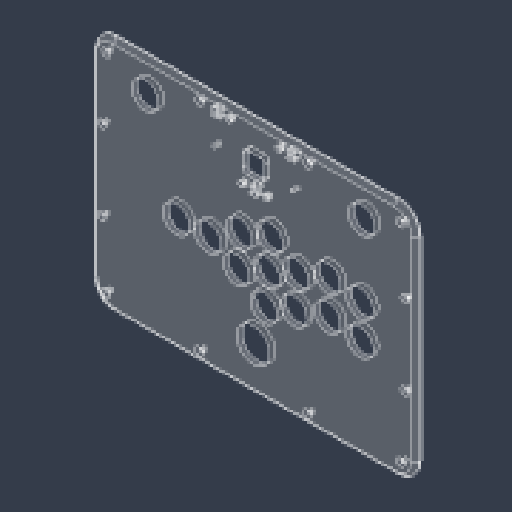
# Autodesk Inventor part: Top Plate Sanwa
Saved by Autodesk Inventor 2023.4 (Build 274418000, 418)
## iProperties
Created: 2024-02-20
Part Number: Top Plate Sanwa
Material: Polycarbonate, Clear
Document SubType Name: Modeling
Designer: JoaoSilva
Density: 1.2 g/cm^3
Appearance: Polycarbonate - Clear
Author: JoaoSilva
Autodesk Inventor part; units mm, degrees
ref_plane "YZ Plane" through (0, 0, 0) normal (1, 0, 0) x (0, 1, 0)
ref_plane "XZ Plane" through (0, 0, 0) normal (0, 1, 0) x (-1, 0, 0)
ref_plane "XY Plane" through (0, 0, 0) normal (0, 0, 1) x (1, 0, 0)
sketch "Sketch1" plane through (0, 0, 0) normal (0, 0, 1) x (1, 0, 0)
  line L0 (-150, 110) -> (150, 110)
  line L1 (150, 110) -> (150, -110)
  line L2 (150, -110) -> (-150, -110)
  line L3 (-150, -110) -> (-150, 110)
  line L4 (-150, 110) -> (150, -110) construction
  line L5 (150, 110) -> (-150, -110) construction
  point P0 (0, 0)
  dimension "d0" = 300
  dimension "d1" = 220
  constraints: 12 end point, 2 midpoint, 2 parallel, 1 horizontal, 1 perpendicular
  measures "d0" distance of L0.start L0.end
  measures "d1" distance of L2.end L0.start
extrude "Extrusion1" add sketch "Sketch1" along normal blind 5
sketch "Sketch2" plane through (0, 0, 5) normal (0, 0, 1) x (1, 0, 0)
  line L0 (-150, -110) -> (150, -110) projected
  line L1 (9.7, -35) -> (14.9, 23.8) construction
  line L2 (-12.9, 12.8) -> (37.5, -24) construction
  line L3 (-100, 80) -> (100, 80) construction
  line L4 (150, 110) -> (-150, 110) projected
  line L5 (-150, 110) -> (-150, -110) projected
  arc A0 (9.7, -35) -> (-41.8, -4.7) centre (-117.4638, -192.22) ccw
  point P0 (0, 0)
  point P1 (0, -70)
  point P2 (-15.5, -17.6)
  point P3 (-71.3, -4.8)
  point P4 (12.3, -5.6)
  point P5 (39.2, 6.1)
  point P6 (68.8, -13.3)
  point P7 (68.8, 17.7)
  point P8 (98.3, -18.3)
  point P9 (98.3, 12.7)
  point P10 (12.3, -5.6)
  point P11 (0, 80)
  point P12 (-60, 80)
  point P13 (60, 80)
  point P14 (31.5334, -55.5137)
  point P15 (-14.9246, -17.9372)
  dimension "d4" = 40
  dimension "d5" = 15.5
  dimension "d6" = 26.3
  dimension "d7" = 29.5
  dimension "d11" = 52.4
  dimension "d12" = 65.3
  dimension "d13" = 65.2
  dimension "d14" = 9.7
  dimension "d15" = 29.4
  dimension "d16" = 2.6
  dimension "d17" = 26.9
  dimension "d18" = 29.6
  dimension "d19" = 29.5
  dimension "d20" = 1.7
  dimension "d22" = 46
  dimension "d23" = 30.1
  dimension "d24" = 96.7
  dimension "d25" = 91.7
  dimension "d26" = 31
  dimension "d27" = 31
  dimension "d28" = 35
  dimension "d61" = 30
  dimension "d62" = 50
  dimension "d63" = 8.496
  dimension "d64" = 8.496
  dimension "d65" = 40
  dimension "d66" = 40
  constraints: 6 end point, 5 point on circle, 4 vertical alignment, 3 midpoint, 2 point on line, 1 centre point, 1 coincident, 1 horizontal
  measures "d4" distance from line of L0 point (0, -70)
  measures "d5" horizontal distance of point (0, -70) point (-15.5, -17.6)
  measures "d6" horizontal distance of A0.end point (-15.5, -17.6)
  measures "d7" horizontal distance of point (-71.3, -4.8) A0.end
  measures "d11" vertical distance of point (0, -70) point (-15.5, -17.6)
  measures "d12" vertical distance of point (0, -70) A0.end
  measures "d13" vertical distance of point (-71.3, -4.8) point (0, -70)
  measures "d14" horizontal distance of L1.start point (0, -70)
  measures "d15" vertical distance of point (12.3, -5.6) L1.start
  measures "d16" horizontal distance of point (12.3, -5.6) L1.start
  measures "d17" horizontal distance of point (39.2, 6.1) point (12.3, -5.6)
  measures "d18" horizontal distance of point (68.8, 17.7) point (39.2, 6.1)
  measures "d19" horizontal distance of point (98.3, 12.7) point (68.8, 17.7)
  measures "d20" horizontal distance of point (39.2, 6.1) L2.end
  measures "d22" vertical distance of L2.end point (0, -70)
  measures "d23" vertical distance of point (39.2, 6.1) L2.end
  measures "d24" distance from line of L0 point (68.8, -13.3)
  measures "d25" distance from line of L0 point (98.3, -18.3)
  measures "d26" distance of point (98.3, 12.7) point (98.3, -18.3)
  measures "d27" distance of point (68.8, -13.3) point (68.8, 17.7)
  measures "d28" vertical distance of L1.start point (0, -70)
  measures "d61" distance between parallel lines of L4 L3
  measures "d62" distance from line of L5 L3.start
  measures "d65" distance of L3.start point (-60, 80)
  measures "d66" distance of L3.end point (60, 80)
hole "Hole1" at (0, -70, 5) at (-15.5, -17.6, 5) at (-41.8, -4.7, 5) at (-71.3, -4.8, 5) at (9.7, -35, 5) at (12.3, -5.6, 5) at (37.5, -24, 5) at (39.2, 6.1, 5) at (68.8, -13.3, 5) at (68.8, 17.7, 5) at (98.3, -18.3, 5) at (98.3, 12.7, 5) at (-12.9, 12.8, 5) at (14.9, 23.8, 5) at (-100, 80, 5) at (100, 80, 5) direction (0, 0, -1) diameter 25 end through all clearance for "Socket Head Cap Screw ISO 4762" size "M24" standard "ISO"
sketch "Sketch5" plane through (0, 0, 5) normal (0, 0, 1) x (1, 0, 0)
  circle A0 centre (0, -70) radius 12.5 projected
  point P0 (0, 0)
hole "Hole2" at (0, -70, 5) direction (0, 0, -1) diameter 31 end through all clearance for "Socket Head Cap Screw ISO 4762" size "M30" standard "ISO"
sketch "Sketch6" plane through (0, 0, 5) normal (0, 0, 1) x (1, 0, 0)
  line L0 (-35.7, 71.2) -> (35.7, 71.2) construction
  line L1 (150, 110) -> (-150, 110) projected
  point P0 (0, 0)
  point P1 (0, 71.2)
  dimension "d67" = 71.4
  dimension "d68" = 38.8
  constraints: 2 end point, 1 horizontal, 1 midpoint, 1 vertical alignment
  measures "d67" distance of L0.start L0.end
  measures "d68" distance between parallel lines of L1 L0
hole "Hole3" at (-35.7, 71.2, 5) at (35.7, 71.2, 5) direction (0, 0, -1) diameter 3.4 end through all clearance for "Socket Head Cap Screw ISO 4762" size "M3" standard "ISO"
fillet "Fillet2" radius 20 4 edges at (-150, 110, 2.5) (-150, -110, 2.5) (150, -110, 2.5) (150, 110, 2.5)
chamfer "Chamfer1" distance 4 angle 45 8 edges at (0, -110, 5) (144.1421, -104.1421, 5) (150, 0, 5) (144.1421, 104.1421, 5) (0, 110, 5) (-144.1421, 104.1421, 5) (-150, 0, 5) (-144.1421, -104.1421, 5)
sketch "Sketch8" plane through (0, 0, 5) normal (0, 0, 1) x (1, 0, 0)
  line L0 (130, 110) -> (-130, 110) projected
  line L1 (-150, 90) -> (-150, -90) projected
  line L2 (-130, -110) -> (130, -110) projected
  line L3 (150, -90) -> (150, 90) projected
  point P0 (0, 0)
  point P1 (-140, 37)
  point P2 (-50, 100)
  point P3 (-136, 96)
  dimension "d85" = 10
  dimension "d86" = 10
  dimension "d87" = 220
  dimension "d88" = 300
  dimension "d89" = 73
  dimension "d90" = 100
  dimension "d91" = 14
  dimension "d92" = 14
  measures "d85" distance from line of L0 point (-50, 100)
  measures "d86" distance from line of L1 point (-140, 37)
  measures "d87" distance between parallel lines of L0 L2
  measures "d88" distance between parallel lines of L3 L1
  measures "d89" distance from line of L0 point (-140, 37)
  measures "d90" distance from line of L1 point (-50, 100)
  measures "d91" distance from line of point (-136, 96) L1
  measures "d92" distance from line of L0 point (-136, 96)
hole "Hole4" at (-140, 37, 5) at (-50, 100, 5) at (-136, 96, 5) direction (0, 0, -1) diameter 3.4 end through all countersink diameter 7.5 countersink angle 90 clearance for "Countersunk Flat Head Hex Socket Screw ISO 10642" size "M3" standard "ISO"
mirror "Mirror1" about plane through (0, 0, 0) normal (1, 0, 0) of "Hole4"
mirror "Mirror2" about plane through (0, 0, 0) normal (0, 1, 0) of "Hole4", "Mirror1"
sketch "Sketch9" plane through (0, 0, 5) normal (0, 0, 1) x (1, 0, 0)
  line L0 (-6, 83.2) -> (6, 83.2)
  line L1 (10, 79.2) -> (10, 67.2)
  line L2 (6, 63.2) -> (-6, 63.2)
  line L3 (-10, 67.2) -> (-10, 79.2)
  circle A0 centre (-35.7, 71.2) radius 1.7 projected
  circle A1 centre (35.7, 71.2) radius 1.7 projected
  line L4 (-35.7, 71.2) -> (35.7, 71.2) construction
  arc A2 (-6, 83.2) -> (-10, 79.2) centre (-6, 79.2) ccw
  arc A3 (10, 79.2) -> (6, 83.2) centre (6, 79.2) ccw
  arc A4 (-10, 67.2) -> (-6, 63.2) centre (-6, 67.2) ccw
  arc A5 (6, 63.2) -> (10, 67.2) centre (6, 67.2) ccw
  point P0 (0, 0)
  point P1 (-10, 83.2)
  point P2 (10, 63.2)
  point P3 (10, 83.2)
  point P4 (0, 83.2)
  point P5 (0, 71.2)
  point P6 (-10, 73.2)
  dimension "d100" = 20
  dimension "d101" = 20
  dimension "d102" = 2
  dimension "d103" = 4
  constraints: 10 end point, 8 point on circle, 8 tangent, 6 point on line, 4 centre point, 3 equal radius, 3 midpoint, 2 horizontal, 2 parallel, 1 perpendicular, 1 vertical alignment
  measures "d100" distance of point (10, 83.2) point (10, 63.2)
  measures "d101" distance of point (-10, 83.2) point (10, 83.2)
  measures "d102" distance from line of L4 point (-10, 73.2)
  measures "d103" radius of A2
extrude "Extrusion5" cut sketch "Sketch9" against normal through all contours L0 A3 L1 A5 L2 A4 L3 A2
sketch "Sketch10" plane through (0, 0, 5) normal (0, 0, 1) x (1, 0, 0)
  line L0 (-11.25, 53.2) -> (11.25, 53.2) construction
  circle A0 centre (35.7, 71.2) radius 1.7 projected
  circle A1 centre (-35.7, 71.2) radius 1.7 projected
  circle A2 centre (35.7, 71.2) radius 1.7 projected
  line L1 (-35.7, 71.2) -> (35.7, 71.2) construction
  line L2 (0, 71.2) -> (0, 98.6) construction
  line L3 (-34.4, 98.6) -> (34.4, 98.6) construction
  line L4 (23.15, 98.6) -> (45.65, 98.6) construction
  line L5 (-45.65, 98.6) -> (-23.15, 98.6) construction
  point P0 (0, 0)
  point P1 (0, 53.2)
  dimension "d106" = 22.5
  dimension "d107" = 18
  dimension "d108" = 22.5
  dimension "d109" = 22.5
  dimension "d110" = 27.4
  dimension "d111" = 68.8
  constraints: 12 end point, 5 horizontal, 5 midpoint, 1 vertical, 1 vertical alignment
  measures "d106" distance of L0.start L0.end
  measures "d107" distance from line of A0.centre L0
  measures "d108" distance of L4.start L4.end
  measures "d109" distance of L5.start L5.end
  measures "d110" distance of L2.start L2.end
  measures "d111" distance of L3.start L3.end
hole "Hole5" at (-11.25, 53.2, 5) at (11.25, 53.2, 5) at (23.15, 98.6, 5) at (-23.15, 98.6, 5) direction (0, 0, -1) diameter 2.9 end through all counterbore diameter 5.5 counterbore depth 2.9 clearance for "Socket Head Cap Screw ISO 4762" size "M2.5" standard "ISO"
sketch "Sketch11" plane through (0, 0, 5) normal (0, 0, 1) x (1, 0, 0)
  circle A0 centre (-11.25, 53.2) radius 1.45 construction
  circle A1 centre (11.25, 53.2) radius 1.45 construction
  line L0 (-11.25, 53.2) -> (11.25, 53.2) construction
  circle A2 centre (23.15, 98.6) radius 1.45 construction
  line L1 (23.15, 98.6) -> (45.65, 98.6) construction
  circle A3 centre (-23.15, 98.6) radius 1.45 construction
  line L2 (-23.15, 98.6) -> (-45.65, 98.6) construction
  line L3 (-2.55, 49.15) -> (2.55, 49.15)
  line L4 (2.55, 49.15) -> (2.55, 57.25)
  line L5 (2.55, 57.25) -> (-2.55, 57.25)
  line L6 (-2.55, 57.25) -> (-2.55, 49.15)
  line L7 (-2.55, 49.15) -> (2.55, 57.25) construction
  line L8 (2.55, 49.15) -> (-2.55, 57.25) construction
  circle A4 centre (-2.55, 50.15) radius 1
  circle A5 centre (2.55, 50.15) radius 1
  circle A6 centre (2.55, 56.25) radius 1
  circle A7 centre (-2.55, 56.25) radius 1
  line L9 (-36.95, 94.55) -> (-31.85, 94.55)
  line L10 (-31.85, 94.55) -> (-31.85, 102.65)
  line L11 (-31.85, 102.65) -> (-36.95, 102.65)
  line L12 (-36.95, 102.65) -> (-36.95, 94.55)
  line L13 (-36.95, 94.55) -> (-31.85, 102.65) construction
  line L14 (-31.85, 94.55) -> (-36.95, 102.65) construction
  circle A8 centre (-36.95, 95.55) radius 1
  circle A9 centre (-31.85, 95.55) radius 1
  circle A10 centre (-31.85, 101.65) radius 1
  circle A11 centre (-36.95, 101.65) radius 1
  line L15 (31.85, 94.55) -> (36.95, 94.55)
  line L16 (36.95, 94.55) -> (36.95, 102.65)
  line L17 (36.95, 102.65) -> (31.85, 102.65)
  line L18 (31.85, 102.65) -> (31.85, 94.55)
  line L19 (31.85, 94.55) -> (36.95, 102.65) construction
  line L20 (36.95, 94.55) -> (31.85, 102.65) construction
  circle A12 centre (31.85, 95.55) radius 1
  circle A13 centre (36.95, 95.55) radius 1
  circle A14 centre (36.95, 101.65) radius 1
  circle A15 centre (31.85, 101.65) radius 1
  point P0 (0, 0)
  point P1 (0, 53.2)
  point P2 (-34.4, 98.6)
  point P3 (34.4, 98.6)
  point P4 (31.85, 100.65)
  point P5 (31.85, 96.55)
  point P6 (36.95, 96.55)
  point P7 (36.95, 100.65)
  point P8 (-31.85, 96.55)
  point P9 (-31.85, 100.65)
  point P10 (-36.95, 100.65)
  point P11 (-36.95, 96.55)
  point P12 (-2.55, 55.25)
  point P13 (-2.55, 51.15)
  point P14 (2.55, 51.15)
  point P15 (2.55, 55.25)
  dimension "d121" = 2
  dimension "d124" = 2
  dimension "d127" = 2
  dimension "d119" = 8.1
  dimension "d120" = 5.1
  dimension "d122" = 8.1
  dimension "d123" = 5.1
  dimension "d125" = 8.1
  dimension "d126" = 5.1
  dimension "d130" = 11.25
  dimension "d131" = 11.25
  dimension "d132" = 11.25
  constraints: 42 end point, 12 point on line, 9 midpoint, 6 horizontal, 6 parallel, 3 perpendicular, 36 other
  measures "d119" distance of L3.end L4.end
  measures "d120" distance of L3.start L3.end
  measures "d122" distance of L10.start L10.end
  measures "d123" distance of L13.start L10.start
  measures "d125" distance of L16.start L16.end
  measures "d126" distance of L19.start L16.start
  measures "d130" distance of point (0, 53.2) L0.start
  measures "d131" distance of L2.start point (-34.4, 98.6)
  measures "d132" distance of L1.start point (34.4, 98.6)
extrude "Extrusion6" cut sketch "Sketch11" against normal through all
equation "\"d64\" = d63"
equation "\"d66\" = d65"
equation "\"d86\" = d85"
equation "\"d90\" = 0.333333 * d88"
equation "\"d92\" = d91"
equation "\"d101\" = d100"
equation "\"d131\" = d130"
equation "\"d132\" = d131"
body "Solid1"
